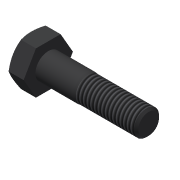
# Autodesk Inventor part: ANSI B18.2.1 - 5/8-11 UNC - 2.5
Saved by Autodesk Inventor 2022 Beta2 (Build 260130000, 130) ContinuousBuild 0
## iProperties
Comments: To add or edit properties for Autodesk Inventor files, use iProperties.
Created: 2003-04-07
Part Number: ANSI B18.2.1 - 5/8-11 UNC - 2.5
Vendor: Autodesk Inc.
Document SubType Name: Modeling
Designer: demo
Description: Heavy Hex Bolt
Standard: ANSI B18.2.1 5/8-11 UNC - 2.5
Density: 1 g/cm^3
Material: Generic
Appearance: Generic
Alert: To add or edit properties for Autodesk Inventor files, use iProperties.
Library Location: C:\Program Files\Autodesk\Inventor 6\content
Library: local
SubLibrary: ANSI
Family: 62
Member: 230
Member Major Revision: 1
Member Minor Revision: 1
Control State: 0
Master: False
Checked Out: False
Shininess: 64.0
Length Units: 11269
Angle Units: 11279
Time Units: 11290
Mass Units: 11283
Length Display Precision: 3
Angle Display Precision: 2
Compacted: True
EGR: 3
Classification: un/spsc 31161513
Density: 0.0
Volumn: 0.0
Area: 0.0
PropertySet Name: Model Information
Author: demo
Revision Number: 1
Autodesk Inventor part; units mm, degrees
ref_plane "YZ Plane" through (0, 0, 0) normal (1, 0, 0) x (0, 1, 0)
ref_plane "XZ Plane" through (0, 0, 0) normal (0, 1, 0) x (-1, 0, 0)
ref_plane "XY Plane" through (0, 0, 0) normal (0, 0, 1) x (1, 0, 0)
sketch "Sketch1" plane through (0, 0, 0) normal (0, 0, 1) x (1, 0, 0)
  line L0 (0, 8.1534) -> (0, 8.1534)
  line L1 (25.4, 7.9375) -> (63.5, 7.9375)
  line L2 (63.5, 7.9375) -> (63.5, 0)
  line L3 (63.5, 0) -> (-0.0001, 0)
  line L4 (-6.3501, 0) -> (82.55, 0) projected
  line L5 (-0.0001, 0) -> (-0.0001, 8.1534)
  line L6 (-0.0001, 8.1534) -> (0, 8.1534)
  line L7 (25.4, 7.9375) -> (24.0258, 8.1534)
  line L8 (24.0258, 8.1534) -> (0, 8.1534)
  line L9 (0, -0.8153) -> (0, 10.5994) projected
  dimension "d0" = 63.5
  dimension "d1" = 38.1
  dimension "d2" = 15.875
  dimension "d9" = 0.0001
  dimension "d10" = 16.3068
  dimension "d13" = 1.3742
  dimension "d14" = 16.3068
  constraints: 16 end point, 3 collinear, 2 perpendicular
  measures "d0" distance between parallel lines of L2 L0
  measures "d1" distance from line of L1.start L2
  measures "d2" diameter of L1 L3
  measures "d9" distance between parallel lines of L5 L0
  measures "d10" diameter of L6 L3
  measures "d13" horizontal distance of L1.start L7.end
  measures "d14" diameter of L8 L3
revolve "Body" add sketch "Sketch1" angle 360 about axis through (63.5, 0, 0) along (-1, 0, 0)
sketch "Sketch2" plane through (-0.0001, 0, 0) normal (-1, 0, 0) x (0, 0, 1)
  line L0 (0, 15.5812) -> (13.4937, 7.7906)
  line L1 (13.4937, 7.7906) -> (13.4937, -7.7906)
  line L2 (13.4937, -7.7906) -> (0, -15.5812)
  line L3 (0, -15.5812) -> (-13.4937, -7.7906)
  line L4 (-13.4937, -7.7906) -> (-13.4937, 7.7906)
  line L5 (-13.4937, 7.7906) -> (0, 15.5812)
  point P0 (0, 0)
  point P1 (0, 0)
  dimension "d11" = 26.9875
  constraints: 12 end point, 1 coincident, 1 vertical, 11 other
  measures "d11" distance between parallel lines of L4 L1
extrude "Head" add sketch "Sketch2" along normal blind 10.7156
sketch "Sketch4" plane through (0, 0, 0) normal (0, 0, 1) x (1, 0, 0)
  line L0 (-10.7157, 13.4938) -> (-10.7157, 15.5812)
  line L1 (-10.7157, 15.5812) -> (-9.5105, 15.5812)
  line L2 (-9.5105, 15.5812) -> (-10.7157, 13.4938)
  line L3 (-11.7873, 0) -> (3.2146, 0) projected
  line L4 (-0.0001, 15.5812) -> (-10.7157, 15.5812) projected
  line L5 (-10.7157, 7.7906) -> (-10.7157, 15.5812) projected
  dimension "d5" = 30
  dimension "d19" = 26.9875
  constraints: 6 end point, 2 collinear, 1 perpendicular, 1 vertical
  measures "d5" angle of L2 L0
  measures "d19" diameter of L0.start L3
revolve "Chamfer1" cut sketch "Sketch4" angle 360 about axis through (-10, 0, 0) along (1, 0, 0)
thread "Thread" size "5/8-11 UNC" class "2A" standard "ANSI Unified Screw Threads" length 38.1
chamfer "Chamfer2" distance 1.3741 distance2 1.3742 1 edges at (63.5, -7.9375, 0) measured on face at (63.5, -0.6813, 3.1515)
equation "\"d0\" = NLG"
equation "\"d1\" = GEL"
equation "\"d2\" = GD"
equation "\"d10\" = SD2"
equation "\"d14\" = BDM"
equation "\"d11\" = SW"
equation "\"d3\" = KOH - SD"
equation "\"d5\" = ANG1"
equation "\"d19\" = SW0"
equation "\"d15\" = GEL"
equation "\"d6\" = -0.5 * SPD + 0.5 * GD"
equation "\"NLG\" = 63.5"
equation "\"GD\" = NND"
equation "\"BDM\" = 16.3068"
equation "\"KOH\" = 10.71562"
equation "\"GEL\" = 38.1"
equation "\"SW\" = 26.9875"
equation "\"SW0\" = SW"
equation "\"SPD\" = 13.12672"
equation "\"SD2\" = BDM"
equation "\"SD\" = 0"
equation "\"ANG1\" = 30deg"
equation "\"GAL\" = GUL"
equation "\"GUL\" = 1.37414"
equation "\"RR\" = 1.524"
equation "\"d20\" = -NLG"
equation "\"TOA\" = 30deg"
equation "\"THREADDIA\" = 15.875"
equation "\"E0\" = 1.155 * SW"
equation "\"GD1\" = SPD"
equation "\"SLG\" = 19.62734"
equation "\"NND\" = 15.875"
body "Solid1"
